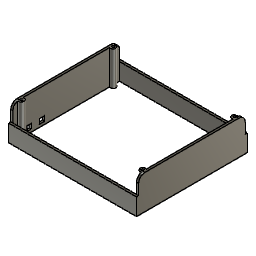
MUS3005Side (Autodesk Fusion 360 design; units mm, degrees)
Autodesk Fusion 360 part; units mm, degrees
sketch "Sketch1" plane through (0, 0, 0) normal (0, 0, 1) x (1, 0, 0)
  line L0 (0, 0) -> (300, 0)
  line L1 (300, 0) -> (300, 260)
  line L2 (300, 260) -> (0, 260)
  line L3 (0, 260) -> (0, 0)
  line L4 (5, 5) -> (295, 5)
  line L5 (295, 5) -> (295, 255)
  line L6 (295, 255) -> (5, 255)
  line L7 (5, 255) -> (5, 5)
  circle A0 centre (7.5, 22.5) radius 2.5
  circle A1 centre (7.5, 237.5) radius 2.5
  circle A2 centre (292.5, 237.5) radius 2.5
  circle A3 centre (292.5, 22.5) radius 2.5
  circle A4 centre (7.5, 237.5) radius 6.5
  circle A5 centre (292.5, 237.5) radius 6.5
  circle A6 centre (292.5, 22.5) radius 6.5
  circle A7 centre (7.5, 22.5) radius 6.5
  dimension "d1" = 300
  dimension "d2" = 260
  dimension "d3" = 290
  dimension "d4" = 250
  dimension "d5" = 5
  dimension "d6" = 5
  dimension "d7" = 5
  dimension "d8" = 5
  dimension "d9" = 5
  dimension "d10" = 5
  dimension "d11" = 5
  dimension "d12" = 5
  dimension "d13" = 22.5
  dimension "d16" = 22.5
  dimension "d17" = 7.5
  dimension "d18" = 7.5
  dimension "d19" = 7.5
  dimension "d20" = 22.5
  dimension "d21" = 7.5
  dimension "d22" = 22.5
  dimension "d23" = 13
  dimension "d24" = 7.5
  dimension "d25" = 22.5
  dimension "d26" = 13
  dimension "d27" = 7.5
  dimension "d28" = 22.5
  dimension "d29" = 13
  dimension "d30" = 7.5
  dimension "d31" = 22.5
  dimension "d32" = 13
  dimension "d33" = 7.5
  dimension "d34" = 22.5
  constraint horizontal L0
  constraint vertical L1
  constraint horizontal L2
  constraint vertical L3
  constraint coincident L0.start L3.end
  constraint horizontal L4
  constraint vertical L5
  constraint horizontal L6
  constraint vertical L7
  measures "d1" distance of L0.start L0.end
  measures "d2" distance of L0.start L2.end
  measures "d3" distance of L4.start L4.end
  measures "d4" distance of L4.start L6.end
  measures "d5" distance of L3 L7
  measures "d6" distance of L0 L4
  measures "d7" distance of L1 L5
  measures "d8" distance of L2 L6
  measures "d9" diameter of A0
  measures "d10" diameter of A1
  measures "d11" diameter of A2
  measures "d12" diameter of A3
  measures "d13" distance of L0 A3.centre
  measures "d16" distance of L2 A2.centre
  measures "d17" distance of L1 A2.centre
  measures "d18" distance of L1 A3.centre
  measures "d19" distance of L3 A0.centre
  measures "d20" distance of L0 A0.centre
  measures "d21" distance of L3 A1.centre
  measures "d22" distance of L2 A1.centre
  measures "d23" diameter of A4
  measures "d24" distance of L3 A1.centre
  measures "d25" distance of L2 A1.centre
  measures "d26" diameter of A5
  measures "d27" distance of L1 A2.centre
  measures "d28" distance of L2 A2.centre
  measures "d29" diameter of A6
  measures "d30" distance of L1 A3.centre
  measures "d31" distance of L0 A3.centre
  measures "d32" diameter of A7
  measures "d33" distance of L3 A0.centre
  measures "d34" distance of L0 A0.centre
extrude "Extrude1" add sketch "Sketch1" along normal blind 80 contours L7 A7 picked at (9.3974, 27.2942) makes body 1
extrude "Extrude2" add sketch "Sketch1" along normal blind 80 separate body contours L5 A6 picked at (287.3448, 22.5) makes body 2
extrude "Extrude3" add sketch "Sketch1" along normal blind 80 separate body contours L5 A5 picked at (287.3448, 237.5) makes body 3
extrude "Extrude4" add sketch "Sketch1" along normal blind 80 separate body contours L7 A4 picked at (9.3974, 242.2942) makes body 4
extrude "Extrude5" add sketch "Sketch1" along normal blind 80 separate body contours L0 L1 L2 L3 makes body 5
extrude "Extrude6" add sketch "Sketch1" along normal blind 80 contours L7 A4 picked at (2.3567, 237.1826) bodies 4 5
extrude "Extrude7" add sketch "Sketch1" along normal blind 80 contours L7 A7 picked at (2.3567, 22.1826) bodies 1 4
extrude "Extrude8" add sketch "Sketch1" along normal blind 80 contours L5 A6 picked at (297.6433, 22.8174) bodies 1 2
extrude "Extrude9" add sketch "Sketch1" along normal blind 80 contours L5 A5 picked at (297.6433, 237.1826) bodies 1 3
sketch "Sketch2" plane through (5, 0, 0) normal (1, 0, 0) x (0, 1, 0)
  line L0 (28.5, 0) -> (231.5, 0)
  line L1 (231.5, 0) -> (231.5, 80)
  line L2 (231.5, 80) -> (28.5, 80)
  line L3 (28.5, 80) -> (28.5, 0)
  line L4 (35, 30) -> (89.718, 30)
  line L5 (89.718, 30) -> (89.718, 0)
  line L6 (89.718, 0) -> (35, 0)
  line L7 (35, 0) -> (35, 30)
  line L8 (5, 0) -> (5, 80)
  line L9 (67.238, 17.75) -> (79.758, 17.75)
  line L10 (79.758, 17.75) -> (79.758, 6.39)
  line L11 (79.758, 6.39) -> (67.238, 6.39)
  line L12 (67.238, 6.39) -> (67.238, 17.75)
  line L13 (38.153, 17.75) -> (48.153, 17.75)
  line L14 (48.153, 17.75) -> (48.153, 6.15)
  line L15 (48.153, 6.15) -> (38.153, 6.15)
  line L16 (38.153, 6.15) -> (38.153, 17.75)
  dimension "d53" = 54.718
  dimension "d56" = 30
  dimension "d57" = 50
  dimension "d58" = 30
  dimension "d59" = 12.52
  dimension "d60" = 10
  dimension "d61" = 9.96
  dimension "d62" = 6.39
  dimension "d63" = 6.15
  dimension "d64" = 19.085
  dimension "d65" = 11.36
  dimension "d66" = 11.6
  constraint horizontal L4
  constraint vertical L5
  constraint horizontal L6
  constraint vertical L7
  constraint horizontal L9
  constraint vertical L10
  constraint horizontal L11
  constraint vertical L12
  constraint horizontal L13
  constraint vertical L14
  constraint horizontal L15
  constraint vertical L16
  measures "d53" distance of L4.start L4.end
  measures "d56" distance of L7 L8
  measures "d57" distance of L2 L4
  measures "d58" distance of L4.start L6.end
  measures "d59" distance of L9.start L9.end
  measures "d60" distance of L13.start L13.end
  measures "d61" distance of L5 L10
  measures "d62" distance of L6 L11
  measures "d63" distance of L6 L15
  measures "d64" distance of L12 L14
  measures "d65" distance of L9.start L11.end
  measures "d66" distance of L13.end L14.end
extrude "Extrude10" cut sketch "Sketch2" against normal blind 5 contours L9 L10 L11 L12 bodies 1
extrude "Extrude11" cut sketch "Sketch2" against normal blind 5 contours L13 L14 L15 L16 bodies 1
sketch "Sketch3" plane through (0, 260, 0) normal (0, 1, 0) x (-1, 0, 0)
  line L0 (-300, 0) -> (0, 0)
  line L1 (0, 0) -> (0, 80)
  line L2 (0, 80) -> (-300, 80)
  line L3 (-300, 80) -> (-300, 0)
  line L4 (-295, 80) -> (-5, 80)
  line L5 (-5, 80) -> (-5, 40)
  line L6 (-5, 40) -> (-295, 40)
  line L7 (-295, 40) -> (-295, 80)
  line L8 (-300, 0) -> (0, 0)
  line L9 (-295, 40) -> (-300, 40)
  line L10 (-300, 40) -> (-300, 80)
  line L11 (-300, 80) -> (-295, 80)
  line L12 (-295, 80) -> (-295, 40)
  line L13 (-5, 40) -> (0, 40)
  line L14 (0, 40) -> (0, 80)
  line L15 (0, 80) -> (-5, 80)
  line L16 (-5, 80) -> (-5, 40)
  dimension "d71" = 290
  dimension "d72" = 5
  dimension "d73" = 5
  dimension "d74" = 40
  dimension "d92" = 5
  dimension "d93" = 40
  dimension "d94" = 5
  dimension "d95" = 40
  constraint horizontal L4
  constraint vertical L5
  constraint horizontal L6
  constraint vertical L7
  constraint coincident L2 L4.start
  constraint horizontal L9
  constraint vertical L10
  constraint horizontal L11
  constraint vertical L12
  constraint horizontal L13
  constraint vertical L14
  constraint horizontal L15
  constraint vertical L16
  measures "d71" distance of L5.end L6.end
  measures "d72" distance of L1 L5
  measures "d73" distance of L3 L7
  measures "d74" distance of L6 L8
  measures "d92" distance of L6.end L9.end
  measures "d93" distance of L9.end L2.end
  measures "d94" distance of L5.end L13.end
  measures "d95" distance of L13.end L1.end
extrude "Extrude12" cut sketch "Sketch3" against normal blind 5 contours L2 L4 L5 L6 L7 L12 L16 bodies 1
sketch "Sketch4" plane through (0, 0, 0) normal (0, -1, 0) x (1, 0, 0)
  line L0 (0, 0) -> (300, 0)
  line L1 (300, 0) -> (300, 80)
  line L2 (300, 80) -> (0, 80)
  line L3 (0, 80) -> (0, 0)
  line L4 (5, 80) -> (295, 80)
  line L5 (295, 80) -> (295, 40)
  line L6 (295, 40) -> (5, 40)
  line L7 (5, 40) -> (5, 80)
  line L8 (0, 0) -> (300, 0)
  line L9 (5, 80) -> (0, 80)
  line L10 (0, 80) -> (0, 40)
  line L11 (0, 40) -> (5, 40)
  line L12 (5, 40) -> (5, 80)
  line L13 (295, 40) -> (300, 40)
  line L14 (300, 40) -> (300, 80)
  line L15 (300, 80) -> (295, 80)
  line L16 (295, 80) -> (295, 40)
  dimension "d77" = 290
  dimension "d78" = 40
  dimension "d79" = 40
  dimension "d80" = 5
  dimension "d81" = 5
  dimension "d84" = 5
  dimension "d85" = 40
  dimension "d86" = 5
  dimension "d87" = 40
  constraint horizontal L4
  constraint vertical L5
  constraint horizontal L6
  constraint vertical L7
  constraint coincident L2 L4.start
  constraint horizontal L9
  constraint vertical L10
  constraint horizontal L11
  constraint vertical L12
  constraint horizontal L13
  constraint vertical L14
  constraint horizontal L15
  constraint vertical L16
  measures "d77" distance of L4.start L4.end
  measures "d78" distance of L4.start L6.end
  measures "d79" distance of L6 L8
  measures "d80" distance of L3 L7
  measures "d81" distance of L1 L5
  measures "d84" distance of L4.start L2.end
  measures "d85" distance of L2.end L10.end
  measures "d86" distance of L5.end L13.end
  measures "d87" distance of L13.end L1.end
extrude "Extrude13" cut sketch "Sketch4" against normal blind 5 contours L2 L4 L5 L6 L7 L12 L16 bodies 1
sketch "Sketch5" plane through (0, 0, 0) normal (-1, 0, 0) x (0, -1, 0)
  line L0 (-48.153, 6.15) -> (-48.153, 17.75)
  line L1 (-48.153, 17.75) -> (-38.153, 17.75)
  line L2 (-38.153, 17.75) -> (-38.153, 6.15)
  line L3 (-38.153, 6.15) -> (-48.153, 6.15)
  line L4 (-79.758, 6.39) -> (-79.758, 17.75)
  line L5 (-79.758, 17.75) -> (-67.238, 17.75)
  line L6 (-67.238, 17.75) -> (-67.238, 6.39)
  line L7 (-67.238, 6.39) -> (-79.758, 6.39)
  line L8 (-260, 0) -> (0, 0)
  line L9 (0, 0) -> (0, 80)
  line L10 (0, 80) -> (-260, 80)
  line L11 (-260, 80) -> (-260, 0)
extrude "Extrude14" cut sketch "Sketch4" against normal blind 5 contours L1 L2 L5 L13 L14 L15 L16 bodies 1
extrude "Extrude15" cut sketch "Sketch4" against normal blind 5 contours L2 L3 L7 L9 L10 L11 L12 bodies 1
extrude "Extrude16" cut sketch "Sketch3" against normal blind 5 contours L1 L2 L5 L13 L14 L15 L16 bodies 1
extrude "Extrude17" cut sketch "Sketch3" against normal blind 5 contours L2 L3 L7 L9 L10 L11 L12 bodies 1
fillet "Fillet1" radius 15 1 edges at (297.5, 5, 80) on bodies 1
fillet "Fillet2" radius 15 1 edges at (297.5, 255, 80) on bodies 1
fillet "Fillet3" radius 15 1 edges at (2.5, 255, 80) on bodies 1
fillet "Fillet4" radius 15 1 edges at (2.5, 5, 80) on bodies 1
